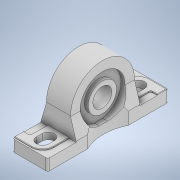
# Autodesk Inventor part: bearing_v2
Saved by Autodesk Inventor 2020 (Build 240168000, 168)
## iProperties
Created: 2022-06-17
Part Number: bearing_v2
Material: 일반
Document SubType Name: Modeling
Designer: samsung
Density: 1 g/cm^3
Appearance: 기본값
Author: samsung
Autodesk Inventor part; units mm, degrees
ref_plane "YZ Plane" through (0, 0, 0) normal (1, 0, 0) x (0, 1, 0)
ref_plane "XZ Plane" through (0, 0, 0) normal (0, 1, 0) x (-1, 0, 0)
sketch "스케치1" plane through (0, 0, 0) normal (0, 1, 0) x (-1, 0, 0)
  line L0 (16.5, -63.5) -> (-16.5, -63.5)
  line L1 (-16.5, 63.5) -> (16.5, 63.5)
  line L2 (18.5, 63.5) -> (-18.5, -63.5) construction
  line L3 (18.5, -63.5) -> (-18.5, 63.5) construction
  line L4 (-13.5, 10) -> (-13.5, -10)
  line L5 (-13.5, -10) -> (13.5, -10)
  line L6 (13.5, -10) -> (13.5, 10)
  line L7 (13.5, 10) -> (-13.5, 10)
  line L8 (-13.5, 10) -> (13.5, -10) construction
  line L9 (-13.5, -10) -> (13.5, 10) construction
  line L10 (18.5, 63.5) -> (-18.5, 63.5)
  line L11 (-18.5, 61.5) -> (-18.5, 21.5)
  line L12 (-18.5, 21.5) -> (18.5, 21.5)
  line L13 (18.5, 21.5) -> (18.5, 63.5)
  line L14 (18.5, -63.5) -> (-18.5, -63.5)
  line L15 (-18.5, -63.5) -> (-18.5, -21.5)
  line L16 (-18.5, -21.5) -> (18.5, -21.5)
  line L17 (18.5, -21.5) -> (18.5, -63.5)
  arc A0 (18.5, 21.5) -> (18.5, -21.5) centre (62.225, 0) ccw
  arc A1 (-18.5, -21.5) -> (-18.5, 21.5) centre (-62.225, 0) ccw
  arc A2 (18.5, 61.5) -> (16.5, 63.5) centre (16.5, 61.5) ccw
  arc A3 (-16.5, 63.5) -> (-18.5, 61.5) centre (-16.5, 61.5) ccw
  arc A4 (-18.5, -61.5) -> (-16.5, -63.5) centre (-16.5, -61.5) ccw
  arc A5 (16.5, -63.5) -> (18.5, -61.5) centre (16.5, -61.5) ccw
  line L18 (18.5, 61.5) -> (18.5, 21.5)
  line L19 (18.5, -21.5) -> (18.5, -61.5)
  line L20 (-18.5, -61.5) -> (-18.5, -21.5)
  line L21 (-18.5, 21.5) -> (-18.5, 63.5)
  point P0 (0, 0)
  dimension "d0" = 127
  dimension "d1" = 37
  dimension "d2" = 20
  dimension "d3" = 27
  dimension "d4" = 42
  dimension "d5" = 42
  dimension "d6" = 2
  constraints: 44 end point, 13 parallel, 12 point on circle, 12 tangent, 6 centre point, 5 perpendicular, 5 point on line, 4 midpoint, 3 equal radius, 2 horizontal, 2 vertical
  measures "d0" distance of L2.start L3.start
  measures "d1" distance of L3.start L2.end
  measures "d2" distance of L4.start L4.end
  measures "d3" distance of L5.end L4.end
  measures "d4" distance of L11.end L10.end
  measures "d5" distance of L14.end L15.end
  measures "d6" radius of A2
extrude "돌출1" add sketch "스케치1" along normal blind 13 contours L0 A4 L15 L16 L17 A5 | L16 A1 L4 L5 L6 A0 | L6 L5 L4 L7 | L6 L7 L4 A1 L12 A0 | L12 L11 A3 L1 A2 L13
sketch "스케치2" plane through (0, 0, 0) normal (0, -1, 0) x (1, 0, 0)
  arc A0 (-18.5, -21.5) -> (-18.5, 21.5) centre (-62.225, 0) ccw projected
  line L0 (-18.5, -61.5) -> (-18.5, -21.5) projected
  arc A1 (-18.5, -61.5) -> (-16.5, -63.5) centre (-16.5, -61.5) ccw projected
  line L1 (16.5, -63.5) -> (-16.5, -63.5) projected
  arc A2 (16.5, -63.5) -> (18.5, -61.5) centre (16.5, -61.5) ccw projected
  line L2 (18.5, -21.5) -> (18.5, -61.5) projected
  arc A3 (18.5, 21.5) -> (18.5, -21.5) centre (62.225, 0) ccw projected
  line L3 (18.5, 61.5) -> (18.5, 21.5) projected
  arc A4 (18.5, 61.5) -> (16.5, 63.5) centre (16.5, 61.5) ccw projected
  line L4 (-16.5, 63.5) -> (16.5, 63.5) projected
  arc A5 (-16.5, 63.5) -> (-18.5, 61.5) centre (-16.5, 61.5) ccw projected
  line L5 (-18.5, 21.5) -> (-18.5, 61.5) projected
  line L6 (18.5, 21.5) -> (-18.5, 21.5)
  line L7 (18.5, -21.5) -> (-18.5, -21.5)
  line L8 (12.5, 55.5) -> (12.5, 29.5)
  line L9 (12.5, -57.5) -> (-12.5, -57.5)
  line L10 (-12.5, -57.5) -> (-12.5, -29.5)
  line L11 (-12.5, 29.5) -> (-12.5, 57.5)
  line L12 (-12.5, 57.5) -> (10.5, 57.5)
  line L13 (10.5, 27.5) -> (-10.5, 27.5)
  line L14 (10.5, -27.5) -> (-10.5, -27.5)
  line L15 (12.5, -29.5) -> (12.5, -57.5)
  line L16 (4.754, -57.5) -> (4.5, -57.5)
  line L17 (4.5, -57.5) -> (4.5, -49.5)
  line L18 (4.5, -49.5) -> (12.5, -49.5)
  line L19 (12.5, -49.5) -> (12.5, -49.754)
  line L20 (-4.754, 57.5) -> (-4.5, 57.5)
  line L21 (-4.5, 57.5) -> (-4.5, 49.5)
  line L22 (-4.5, 49.5) -> (-12.5, 49.5)
  line L23 (-12.5, 49.5) -> (-12.5, 49.754)
  arc A6 (11, -51.6905) -> (6.6905, -56) centre (12.5, -57.5) ccw
  arc A7 (-11, 51.6905) -> (-6.6905, 56) centre (-12.5, 57.5) ccw
  arc A8 (11, -51.6905) -> (12.5, -49.754) centre (10.5, -49.754) ccw
  arc A9 (4.754, -57.5) -> (6.6905, -56) centre (4.754, -55.5) ccw
  arc A10 (-4.754, 57.5) -> (-6.6905, 56) centre (-4.754, 55.5) ccw
  arc A11 (-11, 51.6905) -> (-12.5, 49.754) centre (-10.5, 49.754) ccw
  arc A12 (-12.5, 29.5) -> (-10.5, 27.5) centre (-10.5, 29.5) ccw
  arc A13 (10.5, 27.5) -> (12.5, 29.5) centre (10.5, 29.5) ccw
  arc A14 (12.5, 55.5) -> (10.5, 57.5) centre (10.5, 55.5) ccw
  arc A15 (12.5, -29.5) -> (10.5, -27.5) centre (10.5, -29.5) ccw
  arc A16 (-10.5, -27.5) -> (-12.5, -29.5) centre (-10.5, -29.5) ccw
  point P0 (0, 0)
  point P1 (-6.5, 57.5)
  point P2 (-12.5, 51.5)
  point P3 (6.5, -57.5)
  point P4 (12.5, -51.5)
  dimension "d9" = 6
  dimension "d10" = 6
  dimension "d11" = 6
  dimension "d12" = 6
  dimension "d13" = 6
  dimension "d14" = 6
  dimension "d15" = 6
  dimension "d16" = 6
  dimension "d17" = 8
  dimension "d18" = 8
  dimension "d19" = 8
  dimension "d20" = 8
  dimension "d21" = 12
  dimension "d22" = 12
  dimension "d23" = 2
  dimension "d24" = 2
  constraints: 36 end point, 26 point on circle, 18 tangent, 11 centre point, 8 point on line, 7 equal radius, 5 parallel, 4 horizontal, 3 perpendicular, 2 coincident
  measures "d9" distance between parallel lines of L4 L12
  measures "d10" distance between parallel lines of L13 L6
  measures "d11" distance between parallel lines of L7 L14
  measures "d12" distance between parallel lines of L8 L3
  measures "d13" distance between parallel lines of L5 L11
  measures "d14" distance between parallel lines of L2 L15
  measures "d15" distance between parallel lines of L1 L9
  measures "d16" distance between parallel lines of L0 L10
  measures "d17" distance of L17.end L18.end
  measures "d18" distance of L16.end L17.end
  measures "d19" distance of L21.end L22.end
  measures "d20" distance of L20.end L21.end
  measures "d21" diameter of A6
  measures "d22" diameter of A7
  measures "d23" radius of A8
  measures "d24" radius of A10
extrude "돌출2" cut sketch "스케치2" against normal blind 6 contours L8 A13 L13 A12 L11 L22 L21 L12 A14 | L21 L22 L11 A11 A7 A10 L12 | L9 L17 L18 L15 A8 A6 A9 | L9 L10 A16 L14 A15 L15 L18 L17
fillet "모깎기1" radius 2 19 edges at (-11.9142, 6, 28.0858) (-12.5, 6, 39.627) (-12.0811, 6, 50.9788) (-8.2574, 6, 53.2574) (-5.9788, 6, 57.0811) (2.873, 6, 57.5) (11.9142, 6, 56.9142) (12.5, 6, 42.5) (11.9142, 6, 28.0858) (0, 6, 27.5) (-11.9142, 6, -28.0858) (0, 6, -27.5) (11.9142, 6, -28.0858) (12.5, 6, -39.627) (12.0811, 6, -50.9788) (8.2574, 6, -53.2574) (5.9788, 6, -57.0811) (-3.873, 6, -57.5) (-12.5, 6, -43.5)
sketch "스케치6" plane through (0, 0, 0) normal (1, 0, 0) x (0, 1, 0)
  circle A0 centre (33.3, 0) radius 10
  line L0 (0, 21.5) -> (0, -21.5)
  line L1 (0, -21.5) -> (10, -21.5)
  line L2 (10, 21.5) -> (10, -21.5)
  line L3 (0, 21.5) -> (10, 21.5)
  circle A1 centre (33.3, 0) radius 21.5
  circle A2 centre (33.3, 0) radius 15
  line L4 (67, 21.5) -> (67, -21.5)
  line L5 (10, 21.5) -> (10, 61.5)
  arc A3 (10, -4.3359) -> (10, 4.3359) centre (33.3, 0) ccw
  line L6 (10, 30.7) -> (10, -30.7)
  line L7 (10, -21.5) -> (10, -61.5)
  line L8 (33.3, 33.7) -> (13, 33.7)
  line L9 (13, 61.5) -> (13, 33.7) projected
  line L10 (0, 63.5) -> (13, 63.5) projected
  line L11 (33.3, -33.7) -> (13, -33.7)
  line L12 (13, -61.5) -> (13, -33.7) projected
  line L13 (0, -63.5) -> (13, -63.5) projected
  arc A4 (33.3, -33.7) -> (33.3, 33.7) centre (33.3, 0) ccw
  circle A5 centre (33.3, 0) radius 21.5
  circle A6 centre (33.3, 0) radius 21.5
  point P0 (0, 0)
  point P1 (0, 0)
  point P2 (13, 21.5)
  point P3 (13, -21.5)
  point P4 (13, 27.7579)
  point P5 (13, -27.7579)
  dimension "d44" = 20
  dimension "d45" = 33.3
  dimension "d46" = 43
  dimension "d47" = 30
  dimension "d48" = 67
  dimension "d105" = 29.8
  dimension "d106" = 29.8
  constraints: 22 end point, 7 centre point, 4 coincident, 4 point on circle, 4 point on line, 2 concentric, 2 horizontal, 1 vertical
  measures "d44" diameter of A0
  measures "d45" distance from line of L0 A0.centre
  measures "d46" diameter of A1
  measures "d47" diameter of A2
  measures "d48" distance between parallel lines of L0 L4
  measures "d105" distance between parallel lines of L10 L8
  measures "d106" distance between parallel lines of L13 L11
sketch "스케치9" plane through (0, 13, 0) normal (0, 1, 0) x (1, 0, 0)
  line L0 (18.5, 21.5) -> (18.5, 61.5) projected
  arc A0 (18.5, 61.5) -> (16.5, 63.5) centre (16.5, 61.5) ccw projected
  line L1 (16.5, 63.5) -> (-16.5, 63.5) projected
  arc A1 (-16.5, 63.5) -> (-18.5, 61.5) centre (-16.5, 61.5) ccw projected
  line L2 (-18.5, 61.5) -> (-18.5, 21.5) projected
  arc A2 (-18.5, -21.5) -> (-18.5, 21.5) centre (-62.225, 0) ccw projected
  line L3 (-18.5, -21.5) -> (-18.5, -61.5) projected
  arc A3 (-18.5, -61.5) -> (-16.5, -63.5) centre (-16.5, -61.5) ccw projected
  line L4 (-16.5, -63.5) -> (16.5, -63.5) projected
  arc A4 (16.5, -63.5) -> (18.5, -61.5) centre (16.5, -61.5) ccw projected
  line L5 (18.5, -61.5) -> (18.5, -21.5) projected
  arc A5 (18.5, 21.5) -> (18.5, -21.5) centre (62.225, 0) ccw projected
  line L6 (-12.5, -27.7579) -> (12.5, -27.7579) projected
  line L7 (12.5, 27.7579) -> (12.5, -27.7579) projected
  line L8 (-12.5, 27.7579) -> (12.5, 27.7579) projected
  line L9 (-12.5, -27.7579) -> (-12.5, 27.7579) projected
  line L10 (12.5, 27.7579) -> (18.5, 27.7579)
  line L11 (12.5, -27.7579) -> (18.5, -27.7579)
  line L12 (18.5, -61.5) -> (18.5, -21.5) projected
  line L13 (-12.5, -27.7579) -> (-18.5, -27.7579)
  line L14 (-12.5, 27.7579) -> (-18.5, 27.7579)
  line L15 (-18.5, 61.5) -> (-18.5, 21.5) projected
  line L16 (-18.5, -33.7) -> (18.5, -33.7)
  line L17 (-18.5, 33.7) -> (18.5, 33.7)
  line L18 (-12.5, 33.7) -> (-12.5, -33.7)
  line L19 (-12.5, -29.5) -> (-12.5, -49.754) projected
  line L20 (12.5, -33.7) -> (12.5, 33.7)
  line L21 (12.5, 49.754) -> (12.5, 29.5) projected
  point P0 (0, 0)
  point P1 (18.5, -27.7579)
  dimension "d117" = 29.8
  dimension "d118" = 29.8
  constraints: 16 end point, 16 point on line, 3 horizontal, 1 perpendicular
  measures "d117" distance between parallel lines of L4 L16
  measures "d118" distance between parallel lines of L1 L17
extrude "돌출6" add sketch "스케치9" along normal blind 20.3 contours A5 L5 L11 L7 L10 L0 | L10 L20 L17 L0 | L5 L16 L20 L11 | L9 L13 L3 A2 L2 L14 | L14 L2 L17 L18 | L18 L16 L3 L13
ref_plane "작업 평면1" through (-18.5, 13, 27.7579) normal (0, 0, 1) x (1, 0, 0)
sketch "스케치10" plane through (-18.5, 13, 33.7) normal (0, 0, 1) x (1, 0, 0)
  line L0 (31, 20.3) -> (31, 0) projected
  line L1 (6, 0) -> (6, 20.3) projected
  line L2 (37, 0) -> (35, 0) projected
  line L3 (2, 0) -> (35, 0) projected
  line L4 (2, 0) -> (0, 0) projected
  line L5 (31, 20.3) -> (31, 0) projected
  line L6 (31, 20.3) -> (37, 0)
  line L7 (6, 20.3) -> (0, 0)
  line L8 (37, 0) -> (0, 0) projected
  line L9 (37, 0) -> (37, 20.3) projected
  line L10 (31, 20.3) -> (37, 20.3) projected
  line L11 (6, 20.3) -> (31, 20.3) projected
  line L12 (0, 20.3) -> (6, 20.3) projected
  line L13 (0, 0) -> (0, 20.3) projected
  point P0 (18.5, -13)
  constraints: 4 end point
extrude "돌출7" cut sketch "스케치10" against normal blind 82.05 contours L10 L9 L6 | L7 L13 L12
extrude "돌출8" cut sketch "스케치6" against normal mid plane 182.05 contours A0 | A3 L2 | A1 | A2
sketch "스케치11" plane through (0, 0, 0) normal (1, 0, 0) x (0, 1, 0)
  line L0 (10, -21.5) -> (10, -61.5)
  line L1 (0, -21.5) -> (10, -21.5)
  line L2 (33.3, -30.7) -> (9.0504, -30.7)
  line L3 (0, 21.5) -> (0, -21.5)
  circle A0 centre (33.3, 0) radius 10
  line L4 (10, 21.5) -> (10, -21.5)
  circle A1 centre (33.3, 0) radius 15
  line L5 (10, 30.7) -> (10, -30.7)
  line L6 (33.3, 30.7) -> (10, 30.7)
  circle A2 centre (33.3, 0) radius 21.5
  arc A3 (10, -4.3359) -> (10, 4.3359) centre (33.3, 0) ccw
  line L7 (64, 21.5) -> (64, -21.5)
  arc A4 (33.3, -30.7) -> (33.3, 30.7) centre (33.3, 0) ccw
  line L8 (0, 21.5) -> (10, 21.5)
  line L9 (10, 21.5) -> (10, 61.5)
  point P0 (0, 0)
  point P1 (0, 0)
  point P2 (0, 0)
  point P3 (10, 4.3359)
  dimension "d60" = 20
  dimension "d61" = 33.3
  dimension "d62" = 43
  dimension "d63" = 30
  dimension "d64" = 64
  dimension "d65" = 7
  constraints: 20 end point, 5 centre point, 5 point on line, 4 coincident, 4 point on circle, 2 horizontal, 1 vertical
  measures "d60" diameter of A0
  measures "d61" distance from line of L3 A0.centre
  measures "d62" diameter of A2
  measures "d63" diameter of A1
  measures "d64" distance between parallel lines of L3 L7
  measures "d65" radial gap between concentric circles of A3 A4
extrude "돌출9" add sketch "스케치11" along normal mid plane 17 contours L4 A3 | A2
sketch "스케치12" plane through (0, 0, 0) normal (1, 0, 0) x (0, 1, 0)
  line L0 (10, -21.5) -> (10, -61.5)
  line L1 (0, -21.5) -> (10, -21.5)
  line L2 (33.3, -30.7) -> (9.0504, -30.7)
  line L3 (0, 21.5) -> (0, -21.5)
  circle A0 centre (33.3, 0) radius 10
  line L4 (10, 21.5) -> (10, -21.5)
  circle A1 centre (33.3, 0) radius 15
  line L5 (10, 30.7) -> (10, -30.7)
  line L6 (33.3, 30.7) -> (10, 30.7)
  circle A2 centre (33.3, 0) radius 21.5
  arc A3 (10, -4.3359) -> (10, 4.3359) centre (33.3, 0) ccw
  line L7 (64, 21.5) -> (64, -21.5)
  arc A4 (33.3, -30.7) -> (33.3, 30.7) centre (33.3, 0) ccw
  line L8 (0, 21.5) -> (10, 21.5)
  line L9 (10, 21.5) -> (10, 61.5)
  point P0 (0, 0)
  point P1 (0, 0)
  point P2 (0, 0)
  dimension "d68" = 20
  dimension "d69" = 33.3
  dimension "d70" = 43
  dimension "d71" = 30
  dimension "d72" = 64
  dimension "d73" = 7
  constraints: 20 end point, 5 centre point, 5 point on line, 4 coincident, 4 point on circle, 2 horizontal, 1 vertical
  measures "d68" diameter of A0
  measures "d69" distance from line of L3 A0.centre
  measures "d70" diameter of A2
  measures "d71" diameter of A1
  measures "d72" distance between parallel lines of L3 L7
  measures "d73" radial gap between concentric circles of A3 A4
extrude "돌출10" add sketch "스케치12" along normal blind 12.5 and the other way blind 18.5 contours A1
sketch "스케치13" plane through (0, 13, 0) normal (0, 1, 0) x (1, 0, 0)
  line L0 (18.5, 33.7) -> (18.5, 61.5) projected
  arc A0 (18.5, 61.5) -> (16.5, 63.5) centre (16.5, 61.5) ccw projected
  line L1 (16.5, 63.5) -> (-16.5, 63.5) projected
  arc A1 (-16.5, 63.5) -> (-18.5, 61.5) centre (-16.5, 61.5) ccw projected
  line L2 (-18.5, 61.5) -> (-18.5, 33.7) projected
  line L3 (-18.5, -33.7) -> (-18.5, -61.5) projected
  arc A2 (-18.5, -61.5) -> (-16.5, -63.5) centre (-16.5, -61.5) ccw projected
  line L4 (-16.5, -63.5) -> (16.5, -63.5) projected
  arc A3 (16.5, -63.5) -> (18.5, -61.5) centre (16.5, -61.5) ccw projected
  line L5 (18.5, -61.5) -> (18.5, -33.7) projected
  circle A4 centre (0, 44.5) radius 6.5
  circle A5 centre (0, 50.5) radius 6.5
  line L6 (-6.5, 50.5) -> (-6.5, 44.5)
  line L7 (6.5, 50.5) -> (6.5, 44.5)
  circle A6 centre (0, -44.5) radius 6.5
  circle A7 centre (0, -50.5) radius 6.5
  line L8 (-6.5, -44.5) -> (-6.5, -50.5)
  line L9 (6.5, -44.5) -> (6.5, -50.5)
  line L10 (12.5, -12.2311) -> (8.5, -12.2311) projected
  line L11 (8.5, -12.2311) -> (-8.5, -12.2311) projected
  line L12 (-8.5, -12.2311) -> (-12.5, -12.2311) projected
  line L13 (-12.5, 12.2311) -> (-8.5, 12.2311) projected
  line L14 (-8.5, 12.2311) -> (8.5, 12.2311) projected
  line L15 (8.5, 12.2311) -> (12.5, 12.2311) projected
  line L16 (-12.5, -12.2311) -> (-12.5, -33.7) projected
  line L17 (-12.5, -33.7) -> (-18.5, -33.7) projected
  line L18 (18.5, -33.7) -> (12.5, -33.7) projected
  line L19 (12.5, -33.7) -> (12.5, -12.2311) projected
  line L20 (12.5, 12.2311) -> (12.5, 33.7) projected
  line L21 (12.5, 33.7) -> (18.5, 33.7) projected
  line L22 (-18.5, 33.7) -> (-12.5, 33.7) projected
  line L23 (-12.5, 33.7) -> (-12.5, 12.2311) projected
  point P0 (0, 0)
  point P1 (0, 47.5)
  point P2 (0, -47.5)
  dimension "d78" = 16
  dimension "d79" = 16
  dimension "d82" = 13
  dimension "d83" = 3
  dimension "d84" = 13
  dimension "d85" = 3
  dimension "d86" = 13
  dimension "d87" = 13
  dimension "d88" = 3
  dimension "d89" = 3
  constraints: 8 end point, 8 point on circle, 4 centre point, 2 tangent, 1 parallel, 1 vertical
  measures "d78" distance from line of point (0, 47.5) L1
  measures "d79" distance from line of point (0, -47.5) L4
  measures "d82" diameter of A4
  measures "d83" distance of point (0, 47.5) A4.centre
  measures "d84" diameter of A5
  measures "d85" distance of A5.centre point (0, 47.5)
  measures "d86" diameter of A6
  measures "d87" diameter of A7
  measures "d88" distance of point (0, -47.5) A6.centre
  measures "d89" distance of A7.centre point (0, -47.5)
extrude "돌출11" cut sketch "스케치13" against normal blind 12.5 contours A4 A5 | L6 A5 A4 | A4 A5 L7 | A5 A4 | A4 A5 | A6 A7 | L9 A7 A6 | A6 A7 L8 | A7 A6 | A6 A7
sketch "스케치14" plane through (-18.5, 0, -61.5) normal (-1, 0, 0) x (0, 0, 1)
  line L0 (0, 0) -> (-2, 0) projected
  line L1 (-2, 0) -> (-2, 10)
  line L2 (-2, 0) -> (-2, 13) projected
  line L3 (33.7421, 13) -> (33.7421, 33.3) projected
  line L4 (-2, 10) -> (33.7421, 13)
  line L5 (0, 13) -> (27.8, 13) projected
  line L6 (0, 0) -> (0, 13) projected
  line L7 (0, 0) -> (40, 0) projected
  line L8 (40, 0) -> (40, 13) projected
  line L9 (83, 0) -> (83, 13) projected
  line L10 (83, 0) -> (123, 0) projected
  line L11 (123, 0) -> (123, 13) projected
  line L12 (95.2, 13) -> (123, 13) projected
  line L13 (124.7295, 0) -> (125, 9.9963)
  line L14 (125, 0) -> (125, 13) projected
  line L15 (125, 9.9963) -> (89.2579, 13)
  line L16 (4.5, 13) -> (4.5, 5.3229) projected
  line L17 (32, 0) -> (32, 4) projected
  line L18 (4.5, 8.2556) -> (32, 8.2556)
  line L19 (32, 8.2556) -> (32, 2)
  line L20 (32, 2) -> (4.5, 2)
  line L21 (4.5, 2) -> (4.5, 8.2556)
  line L22 (118.1638, 8.2556) -> (91, 8.2556)
  line L23 (91, 8.2556) -> (91, 2)
  line L24 (91, 2) -> (118.1638, 2)
  line L25 (118.1638, 2) -> (118.1638, 8.2556)
  line L26 (95.2, 13) -> (83, 13) projected
  line L27 (40, 13) -> (27.8, 13) projected
  point P0 (61.5, 0)
  dimension "d92" = 10
  dimension "d93" = 10
  constraints: 24 end point, 5 point on line, 4 parallel, 2 horizontal, 2 perpendicular, 1 midpoint
  measures "d92" distance of L0.end L1.end
  measures "d93" distance of L13.start L13.end
extrude "돌출12" add sketch "스케치14" along normal blind 1 contours L20 L21 L16 L18 L19 L17 | L25 L24 L23 L22
sketch "스케치15" plane through (0, 13, 0) normal (0, 1, 0) x (1, 0, 0)
  line L0 (-6.5, 44.5) -> (-6.5, 50.5) projected
  arc A0 (-6.5, 44.5) -> (6.5, 44.5) centre (0, 44.5) ccw projected
  arc A1 (6.5, 50.5) -> (-6.5, 50.5) centre (0, 50.5) ccw projected
  line L1 (6.5, 50.5) -> (6.5, 44.5) projected
  arc A2 (6.5, -44.5) -> (-6.5, -44.5) centre (0, -44.5) ccw projected
  arc A3 (-6.5, -50.5) -> (6.5, -50.5) centre (0, -50.5) ccw projected
  line L2 (6.5, -44.5) -> (6.5, -50.5) projected
  line L3 (-6.5, -50.5) -> (-6.5, -44.5) projected
  line L4 (-11.5, 44.5) -> (-11.5, 50.5)
  arc A4 (11.5, 50.5) -> (-11.5, 50.5) centre (0, 50.5) ccw
  line L5 (11.5, 50) -> (11.5, 44.5)
  arc A5 (-11.5, -50.5) -> (11.5, -50.5) centre (0, -50.5) ccw
  line L6 (-11.5, -50) -> (-11.5, -44.5)
  line L7 (11.5, -44.5) -> (11.5, -50.5)
  arc A6 (6.5, 50.5) -> (-6.5, 50.5) centre (0, 50.5) ccw projected
  line L8 (6.5, 50.5) -> (6.5, 44.5) projected
  arc A7 (-6.5, 44.5) -> (6.5, 44.5) centre (0, 44.5) ccw projected
  line L9 (-6.5, 44.5) -> (-6.5, 50.5) projected
  line L10 (18.5, 33.7) -> (18.5, 61.5) projected
  arc A8 (18.5, 61.5) -> (16.5, 63.5) centre (16.5, 61.5) ccw projected
  line L11 (16.5, 63.5) -> (-16.5, 63.5) projected
  arc A9 (-16.5, 63.5) -> (-18.5, 61.5) centre (-16.5, 61.5) ccw projected
  line L12 (-18.5, 61.5) -> (-18.5, 33.7) projected
  arc A10 (6.5, -44.5) -> (-6.5, -44.5) centre (0, -44.5) ccw projected
  line L13 (6.5, -44.5) -> (6.5, -50.5) projected
  arc A11 (-6.5, -50.5) -> (6.5, -50.5) centre (0, -50.5) ccw projected
  line L14 (-6.5, -50.5) -> (-6.5, -44.5) projected
  line L15 (-18.5, -33.7) -> (-18.5, -61.5) projected
  arc A12 (-18.5, -61.5) -> (-16.5, -63.5) centre (-16.5, -61.5) ccw projected
  line L16 (-16.5, -63.5) -> (16.5, -63.5) projected
  arc A13 (16.5, -63.5) -> (18.5, -61.5) centre (16.5, -61.5) ccw projected
  line L17 (18.5, -61.5) -> (18.5, -33.7) projected
  line L18 (0, 62) -> (18.4365, 62)
  arc A14 (18.5, 61.5) -> (16.5, 63.5) centre (16.5, 61.5) ccw projected
  line L19 (13.5, 52) -> (18.5, 52)
  line L20 (18.5, 21.5) -> (18.5, 61.5) projected
  line L21 (0, -62) -> (-18.4365, -62)
  line L22 (18.5, 52) -> (18.5, 27.7579)
  line L23 (-18.5, -33.7) -> (-18.5, -61.5) projected
  line L24 (-18.5, -52) -> (-18.5, -27.7579)
  line L25 (-13.5, -52) -> (-18.5, -52)
  arc A15 (13.5, 52) -> (11.5, 50) centre (13.5, 50) ccw
  arc A16 (-13.5, -52) -> (-11.5, -50) centre (-13.5, -50) ccw
  line L26 (12.5, -12.2311) -> (8.5, -12.2311) projected
  line L27 (8.5, -12.2311) -> (-8.5, -12.2311) projected
  line L28 (-8.5, -12.2311) -> (-12.5, -12.2311) projected
  line L29 (-12.5, 12.2311) -> (-8.5, 12.2311) projected
  line L30 (-8.5, 12.2311) -> (8.5, 12.2311) projected
  line L31 (8.5, 12.2311) -> (12.5, 12.2311) projected
  line L32 (-11.5, 44.5) -> (-11.5, 33.7)
  line L33 (11.5, 44.5) -> (11.5, 33.7)
  line L34 (11.5, -44.5) -> (11.5, -33.7)
  line L35 (-11.5, -44.5) -> (-11.5, -33.7)
  line L36 (-12.5, -12.2311) -> (-12.5, -33.7) projected
  line L37 (-12.5, -33.7) -> (-18.5, -33.7) projected
  line L38 (18.5, -33.7) -> (12.5, -33.7) projected
  line L39 (12.5, -33.7) -> (12.5, -12.2311) projected
  line L40 (12.5, 12.2311) -> (12.5, 33.7) projected
  line L41 (12.5, 33.7) -> (18.5, 33.7) projected
  line L42 (-18.5, 33.7) -> (-12.5, 33.7) projected
  line L43 (-12.5, 33.7) -> (-12.5, 12.2311) projected
  line L44 (-12.5, -29.5) -> (-12.5, -33.7)
  line L45 (-18.5, 33.7) -> (18.5, 33.7)
  line L46 (-18.5, 29.5) -> (-18.5, 57) projected
  line L47 (-18.5, -33.7) -> (18.5, -33.7)
  line L48 (18.5, -61.5) -> (18.5, -21.5) projected
  point P0 (0, 0)
  point P1 (11.4018, 52)
  point P2 (-11.4018, -52)
  dimension "d96" = 5
  dimension "d97" = 5
  dimension "d103" = 2
  constraints: 34 end point, 14 point on circle, 9 point on line, 4 centre point, 4 tangent, 3 perpendicular, 2 collinear, 2 horizontal, 2 vertical, 1 equal radius, 3 other
  measures "d96" distance between parallel lines of L1 L5
  measures "d97" radial gap between concentric circles of A3 A5
  measures "d103" radius of A15
extrude "돌출13" cut sketch "스케치15" against normal blind 1 contours L32 L45 L42 L12 A9 L11 A8 L18 A4 L4 | L33 L5 A15 L19 L10 L41 L45 | A5 L7 L34 L47 L38 L17 A13 L16 A12 L21 | L15 L37 L47 L35 L6 A16 L25
fillet "모깎기2" radius 0.5 19 edges at (-18.5, 12.5, 52) (-18.4365, 12.5, 62) (-18.4841, 13, 61.752) (-18.5, 13, 56.75) (-12.0858, 13, 51.4142) (-11.5, 13, 41.85) (-16, 13, 52) (16, 13, -52) (11.5, 13, -41.85) (12.0858, 13, -51.4142) (18.4365, 12.5, -62) (18.4841, 13, -61.752) (18.5, 13, -56.75) (-8.1317, 13, -58.6317) (-11.5, 13, -42.1) (9.2182, 13, -62) (11.5, 13, 42.1) (-9.2182, 13, 62) (8.1317, 13, 58.6317)
sketch "스케치16" plane through (0, 0, 0) normal (1, 0, 0) x (0, 1, 0)
  line L0 (10, -21.5) -> (10, -61.5)
  line L1 (0, -21.5) -> (10, -21.5)
  line L2 (0, 21.5) -> (0, -21.5)
  circle A0 centre (33.3, 0) radius 10
  line L3 (10, 21.5) -> (10, -21.5)
  circle A1 centre (33.3, 0) radius 15
  line L4 (10, 30.7) -> (10, -30.7)
  arc A2 (10, -4.3359) -> (10, 4.3359) centre (33.3, 0) ccw
  line L5 (67, 21.5) -> (67, -21.5)
  line L6 (0, 21.5) -> (10, 21.5)
  line L7 (10, 21.5) -> (10, 61.5)
  line L8 (33.3, 33.7) -> (13, 33.7)
  line L9 (13, 61.5) -> (13, 27.7579)
  line L10 (0, 63.5) -> (13, 63.5)
  line L11 (33.3, -33.7) -> (13, -33.7)
  line L12 (13, -61.5) -> (13, -27.7579)
  line L13 (0, -63.5) -> (13, -63.5)
  arc A3 (33.3, -33.7) -> (33.3, 33.7) centre (33.3, 0) ccw
  line L14 (13, 33.7) -> (13, -33.7)
  line L15 (13, -33.5) -> (13, -44.5) projected
  point P0 (0, 0)
  point P1 (0, 0)
  point P2 (0, 0)
  point P3 (13, 12.2311)
  point P4 (13, -12.2311)
  dimension "d108" = 20
  dimension "d109" = 33.3
  dimension "d111" = 30
  dimension "d112" = 67
  dimension "d113" = 29.8
  dimension "d114" = 29.8
  constraints: 30 end point, 6 point on line, 4 centre point, 4 point on circle, 2 horizontal, 1 collinear, 1 vertical
  measures "d108" diameter of A0
  measures "d109" distance from line of L2 A0.centre
  measures "d111" diameter of A1
  measures "d112" distance between parallel lines of L2 L5
  measures "d113" distance between parallel lines of L10 L8
  measures "d114" distance between parallel lines of L13 L11
extrude "돌출14" add sketch "스케치16" along normal mid plane 25.4 contours A2 L14 L9 L8 A3 L11 L12
